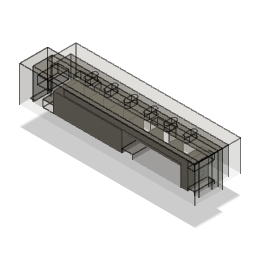
Ramp action bite sensor (Autodesk Fusion 360 design; units mm, degrees)
Autodesk Fusion 360 part; units mm, degrees
note: some values were not read from the file. Chosen so that the rebuilt part matches the saved one: which bodies a step acts on; which face or edge a step refers to. Set by a fixed rule: which sketch regions a step uses.
sketch "Sketch1" plane through (0, 0, 0) normal (0, 0, 1) x (1, 0, 0)
  line L0 (0, 0) -> (19.65, 0)
  line L1 (19.65, 0) -> (19.65, 6.7)
  line L2 (19.65, 6.7) -> (0, 6.7)
  line L3 (0, 6.7) -> (0, 0)
  dimension "d1" = 6.7
  dimension "d2" = 19.65
  constraint horizontal L0
  constraint vertical L1
  constraint horizontal L2
  constraint vertical L3
  constraint coincident L0.start L3.end
  measures "d1" distance of L0.start L2.end
  measures "d2" distance of L1 L3
extrude "Extrude1" add sketch "Sketch1" along normal blind 5.75 makes body 1
sketch "Sketch2" plane through (0, 0, 0) normal (-1, 0, 0) x (0, 0, 1)
  line L0 (0, 6.7) -> (0, 0)
  line L1 (0, 0) -> (5.75, 0)
  line L2 (5.75, 0) -> (5.75, 6.7)
  line L3 (5.75, 6.7) -> (0, 6.7)
  circle A0 centre (1.675, 0.4) radius 0.35
  circle A1 centre (2.875, 0.4) radius 0.35
  circle A2 centre (4.075, 0.4) radius 0.35
  line L4 (1.675, 0.4) -> (2.875, 0.4) construction
  line L5 (2.875, 0.4) -> (4.075, 0.4) construction
  line L6 (2.875, 0) -> (2.875, 1.1832) construction
  dimension "d5" = 0.7
  dimension "d6" = 1.2
  dimension "d7" = 0.4
  constraint equal A0 A1
  constraint equal A1 A2
  constraint coincident A0.centre L4.start
  constraint coincident A1.centre L4.end
  constraint parallel L1 L4
  constraint coincident A2.centre L5.end
  constraint parallel L4 L5
  constraint equal L4 L5
  constraint midpoint L1 L6.start
  constraint perpendicular L5 L6
  constraint coincident A1.centre L6
  measures "d5" diameter of A2
  measures "d6" distance of A0.centre A1.centre
  measures "d7" distance of L1 L5
extrude "Extrude2" add sketch "Sketch2" along normal blind 10 contours A0 | A1 | A2 bodies 1
sketch "Sketch3" plane through (0, 0, 0) normal (-1, 0, 0) x (0, 0, 1)
  circle A0 centre (1.675, 0.4) radius 0.35
  circle A1 centre (4.075, 0.4) radius 0.35
  line L0 (0, 6.7) -> (0, 0)
  line L1 (0, 0) -> (5.75, 0)
  line L2 (5.75, 0) -> (5.75, 6.7)
  line L3 (5.75, 6.7) -> (0, 6.7)
  line L4 (2.875, 6.7) -> (2.875, 2.6069) construction
  circle A2 centre (2.875, 4.5) radius 0.825
  circle A3 centre (2.875, 0.4) radius 0.35
  dimension "d10" = 1.65
  dimension "d11" = 4.5
  constraint midpoint L3 L4.start
  constraint perpendicular L3 L4
  constraint coincident L4 A2.centre
  measures "d10" diameter of A2
  measures "d11" distance of L1 A2.centre
extrude "Extrude3" cut sketch "Sketch3" against normal through all contours A2 bodies 1
sketch "Sketch4" plane through (0, 0, 0) normal (-1, 0, 0) x (0, 0, 1)
  circle A0 centre (2.875, 4.5) radius 0.825
  circle A1 centre (1.675, 0.4) radius 0.35
  circle A2 centre (4.075, 0.4) radius 0.35
  line L0 (0, 6.7) -> (0, 0)
  line L1 (0, 0) -> (5.75, 0)
  line L2 (5.75, 0) -> (5.75, 6.7)
  line L3 (5.75, 6.7) -> (0, 6.7)
  circle A3 centre (2.875, 4.5) radius 0.8
  circle A4 centre (2.875, 0.4) radius 0.35
  dimension "d13" = 1.6
  constraint concentric A0 A3
  measures "d13" diameter of A3
extrude "Extrude4" add sketch "Sketch4" along normal blind 0.4 and the other way blind 40 separate body contours A3 makes body 2
copy_body "Body->Comp1" bodies 1 removing the originals makes body 3 in component "Linear pot body"
copy_body "Body->Comp2" bodies 2 removing the originals makes body 4 in component "Linear pot shaft"
sketch "Sketch5" plane through (0, 0, 0) normal (0, 0, -1) x (-1, 0, 0)
  line L0 (0, 0) -> (0, 6.7)
  line L1 (0, 6.7) -> (-19.65, 6.7)
  line L2 (-19.65, 6.7) -> (-19.65, 0)
  line L3 (-19.65, 0) -> (0, 0)
  line L4 (1, -0.25) -> (1, -1.9)
  line L5 (1, -1.9) -> (-34.65, -1.9)
  line L6 (-34.65, -1.9) -> (-34.65, 8.6)
  line L7 (-34.65, 8.6) -> (1, 8.6)
  line L8 (1, 8.6) -> (1, 6.95)
  line L9 (1, 6.95) -> (-32.65, 6.95)
  line L10 (-32.65, 6.95) -> (-32.65, -0.25)
  line L11 (-32.65, -0.25) -> (1, -0.25)
  dimension "d26" = 0.25
  dimension "d27" = 0.25
  dimension "d28" = 1.65
  dimension "d29" = 1.65
  dimension "d30" = 13
  dimension "d31" = 2
  dimension "d34" = 1
  constraint perpendicular L3 L4
  constraint perpendicular L4 L5
  constraint perpendicular L5 L6
  constraint perpendicular L6 L7
  constraint perpendicular L5 L8
  constraint perpendicular L8 L9
  constraint perpendicular L5 L10
  constraint perpendicular L4 L11
  constraint collinear L4 L8
  measures "d26" distance of L3 L11
  measures "d27" distance of L1 L9
  measures "d28" distance of L5 L11
  measures "d29" distance of L7 L9
  measures "d30" distance of L2 L10
  measures "d31" distance of L6 L10
  measures "d34" distance of L0 L8
extrude "Extrude5" add sketch "Sketch5" against normal up to surface (5.75 mm away) separate body contours L4 L5 L6 L7 L8 L9 L10 L11 makes body 5
sketch "Sketch6" plane through (0, 8.6, 0) normal (0, 1, 0) x (-1, 0, 0)
  line L0 (-34.65, 0) -> (1, 0)
  line L1 (1, 0) -> (1, 5.75)
  line L2 (1, 5.75) -> (-34.65, 5.75)
  line L3 (-34.65, 5.75) -> (-34.65, 0)
  line L4 (1, 0) -> (-3.5, 4.5)
  line L5 (-3.5, 4.5) -> (-4.7, 4.5)
  line L6 (-4.7, 4.5) -> (-4.7, 0)
  line L7 (-4.7, 0) -> (-9.2, 4.5)
  line L8 (-9.2, 4.5) -> (-10.4, 4.5)
  line L9 (-10.4, 4.5) -> (-10.4, 0)
  line L10 (-10.4, 0) -> (-14.9, 4.5)
  line L11 (-14.9, 4.5) -> (-16.1, 4.5)
  line L12 (-16.1, 4.5) -> (-16.1, 0)
  line L13 (-16.1, 0) -> (-20.6, 4.5)
  line L14 (-20.6, 4.5) -> (-21.8, 4.5)
  line L15 (-21.8, 4.5) -> (-21.8, 0)
  line L16 (-21.8, 0) -> (-26.3, 4.5)
  line L17 (-26.3, 4.5) -> (-27.5, 4.5)
  line L18 (-27.5, 4.5) -> (-27.5, 0)
  line L19 (-27.5, 0) -> (-31.829, 4.329)
  line L20 (-31.829, 4.329) -> (-33.029, 4.329)
  line L21 (-33.029, 4.329) -> (-33.029, 0)
  dimension "d35" = 4.5
  dimension "d36" = 135
  dimension "d38" = 1.2
  dimension "d42" = 1.2
  dimension "d58" = 5.7
  constraint coincident L0.end L1.start
  constraint perpendicular L1 L5
  constraint coincident L0 L6.end
  constraint perpendicular L0 L6
  constraint perpendicular L6 L8
  constraint coincident L0 L9.end
  constraint perpendicular L0 L9
  constraint perpendicular L9 L11
  constraint coincident L0 L12.end
  constraint perpendicular L0 L12
  constraint parallel L10 L13
  constraint perpendicular L12 L14
  constraint coincident L0 L15.end
  constraint perpendicular L0 L15
  constraint parallel L13 L16
  constraint perpendicular L15 L17
  constraint coincident L0 L18.end
  constraint perpendicular L0 L18
  constraint collinear L5 L8
  constraint collinear L8 L11
  constraint collinear L11 L14
  constraint collinear L14 L17
  constraint equal L5 L8
  constraint equal L8 L11
  constraint equal L11 L14
  constraint equal L14 L17
  constraint parallel L7 L10
  constraint parallel L4 L7
  constraint perpendicular L18 L20
  constraint coincident L0 L21.end
  constraint perpendicular L0 L21
  constraint parallel L16 L19
  measures "d35" distance of L0 L5
  measures "d36" angle of L4 L5
  measures "d38" distance of L4.end L5.end
  measures "d42" distance of L19.end L20.end
  measures "d58" distance of L0.end L6.end
extrude "Extrude6" cut sketch "Sketch6" against normal through all contours L0 L19 L20 L21 | L0 L16 L17 L18 | L0 L13 L14 L15 | L0 L4 L5 L6 | L0 L10 L11 L12 | L0 L7 L8 L9 bodies 5
sketch "Sketch7" plane through (0, 0, 0) normal (0, 0, -1) x (-1, 0, 0)
  line L0 (0, 0) -> (0, 6.7)
  line L1 (0, 6.7) -> (-19.65, 6.7)
  line L2 (-19.65, 6.7) -> (-19.65, 0)
  line L3 (-19.65, 0) -> (0, 0)
  line L4 (4.7, 8.75) -> (-40.7, 8.75)
  line L5 (-40.7, 8.75) -> (-40.7, -2.05)
  line L6 (-40.7, -2.05) -> (4.7, -2.05)
  line L7 (4.7, -2.05) -> (4.7, 8.75)
  line L8 (-27.5, 8.6) -> (-26.3, 8.6)
  line L9 (-21.8, -1.9) -> (-26.3, -1.9)
  line L10 (4.2, 3.7) -> (4.2, 5.3)
  line L11 (-36.2, 5.3) -> (-36.2, 3.7)
  line L12 (-41.7, -3.05) -> (5.7, -3.05)
  line L13 (5.7, -3.05) -> (5.7, 9.75)
  line L14 (5.7, 9.75) -> (-41.7, 9.75)
  line L15 (-41.7, 9.75) -> (-41.7, -3.05)
  dimension "d44" = 0.15
  dimension "d45" = 0.15
  dimension "d46" = 0.5
  dimension "d47" = 4.5
  dimension "d48" = 1
  constraint horizontal L4
  constraint vertical L5
  constraint horizontal L6
  constraint vertical L7
  measures "d44" distance of L4 L8
  measures "d45" distance of L6 L9
  measures "d46" distance of L7 L10
  measures "d47" distance of L5 L11
extrude "Extrude7" add sketch "Sketch7" along normal blind 2.5 and the other way up to surface (5.75 mm away) separate body contours L12 L13 L14 L15 makes body 6
sketch "Sketch8" plane through (0, 8.75, 0) normal (0, -1, 0) x (1, 0, 0)
  line L0 (-4.7, 5.75) -> (-4.7, -2.5)
  line L1 (-4.7, -2.5) -> (40.7, -2.5)
  line L2 (40.7, -2.5) -> (40.7, 5.75)
  line L3 (40.7, 5.75) -> (-4.7, 5.75)
  circle A0 centre (32.2034, 3.5144) radius 0.75
  line L4 (32.2034, 3.5144) -> (32.2034, 1.5144) construction
  circle A1 centre (32.2034, 1.5144) radius 0.75
  line L5 (31.4534, 1.5144) -> (31.4534, 3.5144)
  line L6 (32.9534, 3.5144) -> (32.9534, 1.5144)
  dimension "d54" = 1.5
  dimension "d55" = 2
  constraint coincident A0.centre L4.start
  constraint perpendicular L1 L4
  constraint coincident L4.end A1.centre
  constraint equal A0 A1
  constraint coincident A0 L5.end
  constraint tangent A0 L5
  constraint tangent A1 L6
  constraint tangent A0 L6
  constraint coincident A0 L6.start
  constraint coincident A1 L5.start
  constraint tangent A1 L5
  constraint coincident A1 L6.end
  measures "d54" diameter of A0
  measures "d55" distance of A0.centre L4.end
extrude "Extrude8" add sketch "Sketch8" along normal blind 1.5 contours A0 | A0 A1 L5 L6 | A1 bodies 5 6
extrude "Extrude9" add sketch "Sketch8" against normal blind 1.75 from surface at 10.8 contours A0 | A0 A1 L5 L6 | A1 bodies 6
pattern_linear "R-Pattern1" count 6 spacing 5.7 along (-1, 0, 0) of "Extrude9"
pattern_linear "R-Pattern2" count 6 spacing 5.7 along (-1, 0, 0) of "Extrude8"
copy_body "Body->Comp3" bodies 6 removing the originals makes body 7 in component "Upper shell"
copy_body "Body->Comp5" bodies 5 removing the originals makes body 8 in component "Slider"
ref_plane "WorkPlane1" through (31.4534, 8, 3.5144) normal (-0.707107, 0, 0.707107) x (0, -1, 0) in component "Upper shell"
sketch "Sketch1 (2)" plane through (31.4534, 8, 3.5144) normal (-0.707107, 0, 0.707107) x (0, -1, 0) in component "Upper shell"
  line L0 (0, 0) -> (0, 0.75) construction
  dimension "d111" = 0.75
  constraint coincident L0.start origin
  constraint vertical L0
  measures "d111" distance of L0.start L0.end
sketch "Sketch2 (2)" plane through (0, 0, -2.5) normal (0, 0, -1) x (-1, 0, 0) in component "Upper shell"
  line L0 (4.7, 8.75) -> (4.7, -2.05)
  line L1 (4.7, -2.05) -> (-40.7, -2.05)
  line L2 (-40.7, -2.05) -> (-40.7, 8.75)
  line L3 (-40.7, 8.75) -> (4.7, 8.75)
  line L4 (-41.7, 9.75) -> (-41.7, -3.05)
  line L5 (-41.7, -3.05) -> (5.7, -3.05)
  line L6 (5.7, -3.05) -> (5.7, 9.75)
  line L7 (5.7, 9.75) -> (-41.7, 9.75)
extrude "Extrude1'" add sketch "Sketch2 (2)" against normal blind 2.5 contours L0 L1 L2 L3 bodies 7 in component "Upper shell"
sketch "Sketch9" plane through (0.75, 0, 5.75) normal (0, 0, 1) x (1, 0, 0)
  line L0 (-0.75, 6.95) -> (32.9, 6.95)
  line L1 (32.9, 6.95) -> (32.9, -0.25)
  line L2 (32.9, -0.25) -> (-0.75, -0.25)
  line L3 (-0.75, -0.25) -> (-0.75, -1.9)
  line L4 (-0.75, -1.9) -> (34.9, -1.9)
  line L5 (34.9, -1.9) -> (34.9, 8.6)
  line L6 (34.9, 8.6) -> (-0.75, 8.6)
  line L7 (-0.75, 8.6) -> (-0.75, 6.95)
  line L8 (39.95, -2.05) -> (-5.45, -2.05)
  line L9 (-5.45, -2.05) -> (-5.45, 8.75)
  line L10 (-5.45, 8.75) -> (39.95, 8.75)
  line L11 (39.95, 8.75) -> (39.95, -2.05)
  line L12 (-6.45, -3.05) -> (40.95, -3.05)
  line L13 (40.95, -3.05) -> (40.95, 9.75)
  line L14 (40.95, 9.75) -> (-6.45, 9.75)
  line L15 (-6.45, 9.75) -> (-6.45, -3.05)
extrude "Extrude10" add sketch "Sketch9" along normal blind 2.5 from surface at 0.02 separate body contours L0 L1 L2 L3 L4 L5 L6 L7 | L8 L9 L10 L11 | L12 L13 L14 L15 makes body 9
copy_body "Body->Comp6" bodies 9 removing the originals makes body 10 in component "Lower shell"
sketch "Sketch1 (3)" plane through (0, 0, 5.77) normal (0, 0, -1) x (-1, 0, 0) in component "Lower shell"
  line L0 (5.7, -3.05) -> (5.7, 9.75)
  line L1 (5.7, 9.75) -> (-41.7, 9.75)
  line L2 (-41.7, 9.75) -> (-41.7, -3.05)
  line L3 (-41.7, -3.05) -> (5.7, -3.05)
  line L4 (0.05, 3.1259) -> (3.05, 3.1259)
  line L5 (3.05, 3.1259) -> (3.05, 1.1259)
  line L6 (3.05, 1.1259) -> (0.05, 1.1259)
  line L7 (0.05, 1.1259) -> (0.05, 3.1259)
  line L8 (0, 6.7) -> (0, 0)
  line L9 (-19.7, 0.3387) -> (-22.8085, 0.3387)
  line L10 (-22.8085, 0.3387) -> (-22.8085, 2.2038)
  line L11 (-22.8085, 2.2038) -> (-19.7, 2.2038)
  line L12 (-19.7, 2.2038) -> (-19.7, 0.3387)
  line L13 (-19.65, 0) -> (-19.65, 6.7)
  dimension "d129" = 0.05
  dimension "d130" = 3
  dimension "d131" = 2
  dimension "d143" = 0.05
  constraint horizontal L4
  constraint vertical L5
  constraint horizontal L6
  constraint vertical L7
  constraint horizontal L9
  constraint vertical L10
  constraint horizontal L11
  constraint vertical L12
  measures "d129" distance of L7 L8
  measures "d130" distance of L5 L7
  measures "d131" distance of L4 L6
  measures "d143" distance of L12 L13
extrude "Extrude1''" add sketch "Sketch1 (3)" along normal up to surface (7.27 mm away) contours L4 L5 L6 L7 | L9 L10 L11 L12 bodies 10 in component "Lower shell"
sketch "Sketch2 (3)" plane through (-0.05, 0, 0) normal (1, 0, 0) x (0, 0, -1) in component "Lower shell"
  line L0 (1.5, 1.1259) -> (1.5, 3.1259)
  line L1 (1.5, 3.1259) -> (-5.77, 3.1259)
  line L2 (-5.77, 3.1259) -> (-5.77, 1.1259)
  line L3 (-5.77, 1.1259) -> (1.5, 1.1259)
  line L4 (1.5, 1.1259) -> (0, 1.1259)
  line L5 (0, 1.1259) -> (0, 3.1259)
  line L6 (0, 3.1259) -> (1.5, 3.1259)
  line L7 (1.5, 3.1259) -> (1.5, 1.1259)
  dimension "d134" = 1.5
  constraint horizontal L4
  constraint vertical L5
  constraint horizontal L6
  constraint vertical L7
  constraint coincident L1 L5.end
  constraint coincident L0.start L3.end
  measures "d134" distance of L5 L7
extrude "Extrude2'" add sketch "Sketch2 (3)" along normal blind 1.2 contours L0 L1 L3 L4 L5 L6 L7 bodies 10 in component "Lower shell"
sketch "Sketch3 (2)" plane through (0, 0, -2.5) normal (0, 0, -1) x (-1, 0, 0) in component "Upper shell"
  line L0 (-41.7, 9.75) -> (-41.7, -3.05)
  line L1 (-41.7, -3.05) -> (5.7, -3.05)
  line L2 (5.7, -3.05) -> (5.7, 9.75)
  line L3 (5.7, 9.75) -> (-41.7, 9.75)
  line L4 (-2.0163, 4.007) -> (3.8111, 4.007)
  line L5 (3.8111, 4.007) -> (3.8111, 0.2402)
  line L6 (3.8111, 0.2402) -> (-2.0163, 0.2402)
  line L7 (-2.0163, 0.2402) -> (-2.0163, 4.007)
  line L8 (-23.5837, 3.4089) -> (-18.248, 3.4089)
  line L9 (-18.248, 3.4089) -> (-18.248, -0.2119)
  line L10 (-18.248, -0.2119) -> (-23.5837, -0.2119)
  line L11 (-23.5837, -0.2119) -> (-23.5837, 3.4089)
  constraint horizontal L4
  constraint vertical L5
  constraint horizontal L6
  constraint vertical L7
  constraint horizontal L8
  constraint vertical L9
  constraint horizontal L10
  constraint vertical L11
extrude "Extrude2''" cut sketch "Sketch3 (2)" against normal through all from surface at -0.5 contours L4 L5 L6 L7 | L8 L9 L10 L11 bodies 7 in component "Upper shell"
sketch "Sketch3 (3)" plane through (0, 0, 5.77) normal (0, 0, -1) x (-1, 0, 0) in component "Lower shell"
  line L0 (3.05, 3.1259) -> (3.05, 1.1259)
  line L1 (3.05, 1.1259) -> (0.05, 1.1259)
  line L2 (0.05, 1.1259) -> (0.05, 3.1259)
  line L3 (0.05, 3.1259) -> (3.05, 3.1259)
  line L4 (5.7, -3.05) -> (5.7, 9.75)
  line L5 (5.7, 9.75) -> (-41.7, 9.75)
  line L6 (-41.7, 9.75) -> (-41.7, -3.05)
  line L7 (-41.7, -3.05) -> (5.7, -3.05)
  line L8 (4.55, 8.4492) -> (1.3881, 8.4492)
  line L9 (1.3881, 8.4492) -> (1.3881, 6.0241)
  line L10 (1.3881, 6.0241) -> (4.55, 6.0241)
  line L11 (4.55, 6.0241) -> (4.55, 8.4492)
  line L12 (4.55, -1.8262) -> (1.3881, -1.8262)
  line L13 (1.3881, -1.8262) -> (1.3881, -0.1246)
  line L14 (1.3881, -0.1246) -> (4.55, -0.1246)
  line L15 (4.55, -0.1246) -> (4.55, -1.8262)
  line L16 (-40.55, 8.4885) -> (-38.5504, 8.4885)
  line L17 (-38.5504, 8.4885) -> (-38.5504, 6.8746)
  line L18 (-38.5504, 6.8746) -> (-40.55, 6.8746)
  line L19 (-40.55, 6.8746) -> (-40.55, 8.4885)
  line L20 (-40.55, -1.7379) -> (-38.5504, -1.7379)
  line L21 (-38.5504, -1.7379) -> (-38.5504, 1.7763)
  line L22 (-38.5504, 1.7763) -> (-40.55, 1.7763)
  line L23 (-40.55, 1.7763) -> (-40.55, -1.7379)
  line L24 (-40.7, -2.05) -> (-40.7, 8.75)
  line L25 (4.7, 8.75) -> (4.7, -2.05)
  line L26 (-22.8085, 0.3387) -> (-22.8085, 2.2038)
  line L27 (-22.8085, 2.2038) -> (-19.7, 2.2038)
  line L28 (-19.7, 2.2038) -> (-19.7, 0.3387)
  line L29 (-19.7, 0.3387) -> (-22.8085, 0.3387)
  dimension "d139" = 0.15
  dimension "d140" = 0.15
  constraint horizontal L8
  constraint vertical L9
  constraint horizontal L10
  constraint vertical L11
  constraint horizontal L12
  constraint vertical L13
  constraint horizontal L14
  constraint vertical L15
  constraint horizontal L16
  constraint vertical L17
  constraint horizontal L18
  constraint vertical L19
  constraint horizontal L20
  constraint vertical L21
  constraint horizontal L22
  constraint vertical L23
  constraint collinear L17 L21
  constraint collinear L19 L23
  constraint collinear L11 L15
  constraint collinear L9 L13
  measures "d139" distance of L23 L24
  measures "d140" distance of L11 L25
extrude "Extrude3'" add sketch "Sketch3 (3)" along normal blind 5.8 contours L8 L9 L10 L11 | L12 L13 L14 L15 | L16 L17 L18 L19 | L20 L21 L22 L23 bodies 10 in component "Lower shell"
sketch "Sketch4 (2)" plane through (19.7, 0, 0) normal (-1, 0, 0) x (0, 0, 1) in component "Lower shell"
  line L0 (-1.5, 2.2038) -> (-1.5, 0.3387)
  line L1 (-1.5, 0.3387) -> (5.77, 0.3387)
  line L2 (5.77, 0.3387) -> (5.77, 2.2038)
  line L3 (5.77, 2.2038) -> (-1.5, 2.2038)
  line L4 (-1.5, 0.3387) -> (-0.05, 0.3387)
  line L5 (-0.05, 0.3387) -> (-0.05, 2.2038)
  line L6 (-0.05, 2.2038) -> (-1.5, 2.2038)
  line L7 (-1.5, 2.2038) -> (-1.5, 0.3387)
  line L8 (0, 0) -> (0, 6.7)
  dimension "d144" = 0.05
  constraint horizontal L4
  constraint vertical L5
  constraint horizontal L6
  constraint vertical L7
  constraint coincident L3 L5.end
  constraint coincident L0.end L1.start
  measures "d144" distance of L5 L8
extrude "Extrude4'" add sketch "Sketch4 (2)" along normal blind 1 contours L0 L1 L3 L4 L5 L6 L7 bodies 10 in component "Lower shell"
chamfer "Chamfer1" distance 1 angle 45 2 edges at (18.7, 1.2712, -1.5) (1.15, 2.1259, -1.5) on bodies 10 in component "Lower shell"
sketch "Sketch4 (3)" plane through (-5.7, 0, 0) normal (-1, 0, 0) x (0, 0, 1) in component "Upper shell"
  line L0 (5.75, 9.75) -> (-2.5, 9.75)
  line L1 (-2.5, 9.75) -> (-2.5, -3.05)
  line L2 (-2.5, -3.05) -> (5.75, -3.05)
  line L3 (5.75, -3.05) -> (5.75, 9.75)
  circle A0 centre (1.8509, 0.4011) radius 0.5
  line L4 (1.8509, 0.9011) -> (6.1961, 0.9011)
  line L5 (1.8509, -0.0989) -> (6.1961, -0.0989)
  line L6 (6.1961, -0.0989) -> (6.1961, 0.9011)
  dimension "d148" = 1
  constraint coincident A0 L4.start
  constraint perpendicular L3 L4
  constraint coincident A0 L5.start
  constraint perpendicular L3 L5
  constraint perpendicular L4 L6
  constraint tangent A0 L4
  constraint tangent A0 L5
  measures "d148" diameter of A0
extrude "Extrude3''" cut sketch "Sketch4 (3)" against normal blind 1.6 contours L3 A0 L4 L5 | A0 bodies 7 in component "Upper shell"
sketch "Sketch5 (2)" plane through (0, 0, 8.27) normal (0, 0, 1) x (1, 0, 0) in component "Lower shell"
  line L0 (-5.7, 9.75) -> (-5.7, -3.05)
  line L1 (-5.7, -3.05) -> (41.7, -3.05)
  line L2 (41.7, -3.05) -> (41.7, 9.75)
  line L3 (41.7, 9.75) -> (-5.7, 9.75)
  line L4 (-5.9, -3.25) -> (41.9, -3.25)
  line L5 (41.9, -3.25) -> (41.9, 9.95)
  line L6 (41.9, 9.95) -> (-5.9, 9.95)
  line L7 (-5.9, 9.95) -> (-5.9, -3.25)
  line L8 (-7.2, -4.55) -> (43.2, -4.55)
  line L9 (43.2, -4.55) -> (43.2, 11.25)
  line L10 (43.2, 11.25) -> (-7.2, 11.25)
  line L11 (-7.2, 11.25) -> (-7.2, -4.55)
  dimension "d151" = 0.2
  dimension "d152" = 1.5
extrude "Extrude5'" add sketch "Sketch5 (2)" against normal up to surface (2.5 mm away) contours L4 L5 L6 L7 bodies 10 in component "Lower shell"
extrude "Extrude6'" add sketch "Sketch5 (2)" against normal blind 8 contours L8 L9 L10 L11 bodies 10 in component "Lower shell"
sketch "Sketch6 (2)" plane through (-7.2, 0, 0) normal (-1, 0, 0) x (0, 0, 1) in component "Lower shell"
  line L0 (8.27, -4.55) -> (8.27, 11.25)
  line L1 (8.27, 11.25) -> (0.27, 11.25)
  line L2 (0.27, 11.25) -> (0.27, -4.55)
  line L3 (0.27, -4.55) -> (8.27, -4.55)
  circle A0 centre (5.1839, 0.3732) radius 0.6326
  line L4 (5.1839, 0.3732) -> (5.1839, 1.0059) construction
  line L5 (5.1839, 0.3732) -> (5.1839, -0.2594) construction
  line L6 (5.1839, 1.0059) -> (-0.3685, 1.0059)
  line L7 (-0.3685, 1.0059) -> (-0.3685, -0.2594)
  line L8 (-0.3685, -0.2594) -> (5.1839, -0.2594)
  constraint coincident A0.centre L4.start
  constraint coincident A0 L4.end
  constraint vertical L4
  constraint coincident A0 L5.end
  constraint parallel L4 L5
  constraint tangent A0 L6
  constraint perpendicular L6 L7
  constraint tangent A0 L8
extrude "Extrude7'" cut sketch "Sketch6 (2)" against normal blind 1.5 contours L2 L6 L7 L8 | L2 A0 L6 L8 | A0 bodies 10 in component "Lower shell"
sketch "Sketch1 (4)" plane through (33.029, 0, 0) normal (-1, 0, 0) x (0, 0, 1) in component "Slider"
  line L0 (0, -1.9) -> (4.329, -1.9)
  line L1 (4.329, -1.9) -> (4.329, 8.6)
  line L2 (4.329, 8.6) -> (0, 8.6)
  line L3 (0, 8.6) -> (0, -1.9)
  circle A0 centre (2.875, 4.5) radius 0.8
  circle A1 centre (2.875, 4.5) radius 0.85
  dimension "d159" = 1.7
  constraint concentric A0 A1
  measures "d159" diameter of A1
extrude "Extrude1'''" cut sketch "Sketch1 (4)" against normal through all contours A0 | A1 bodies 8 in component "Slider"
sketch "Sketch10" plane through (0, 0, 8.27) normal (0, 0, 1) x (1, 0, 0)
  line L0 (-7.2, 11.25) -> (-7.2, -4.55)
  line L1 (-7.2, -4.55) -> (43.2, -4.55)
  line L2 (43.2, -4.55) -> (43.2, 11.25)
  line L3 (43.2, 11.25) -> (-7.2, 11.25)
  line L4 (-7.7, -5.05) -> (43.7, -5.05)
  line L5 (43.7, -5.05) -> (43.7, 11.75)
  line L6 (43.7, 11.75) -> (-7.7, 11.75)
  line L7 (-7.7, 11.75) -> (-7.7, -5.05)
  line L8 (-9.05, -6.4) -> (45.05, -6.4)
  line L9 (45.05, -6.4) -> (45.05, 13.1)
  line L10 (45.05, 13.1) -> (-9.05, 13.1)
  line L11 (-9.05, 13.1) -> (-9.05, -6.4)
  dimension "d161" = 0.5
  dimension "d162" = 1.85
extrude "Extrude11" add sketch "Sketch10" against normal blind 7.5 separate body contours L8 L9 L10 L11 makes body 11
sketch "Sketch11" plane through (0, 0, 8.27) normal (0, 0, 1) x (1, 0, 0)
  line L0 (-7.7, -5.05) -> (-7.7, 11.75)
  line L1 (-7.7, 11.75) -> (43.7, 11.75)
  line L2 (43.7, 11.75) -> (43.7, -5.05)
  line L3 (43.7, -5.05) -> (-7.7, -5.05)
  line L4 (-9.05, 13.1) -> (-9.05, -6.4)
  line L5 (-9.05, -6.4) -> (45.05, -6.4)
  line L6 (45.05, -6.4) -> (45.05, 13.1)
  line L7 (45.05, 13.1) -> (-9.05, 13.1)
extrude "Extrude12" add sketch "Sketch11" along normal blind 2.25 contours L0 L1 L2 L3 | L4 L5 L6 L7 bodies 11
fillet "Fillet1" radius 1.5 8 edges at (-9.05, 13.1, 5.645) (18, 13.1, 10.52) (-9.05, 3.35, 10.52) (45.05, 3.35, 10.52) (45.05, 13.1, 5.645) (18, -6.4, 10.52) (45.05, -6.4, 5.645) (-9.05, -6.4, 5.645) on bodies 11
sketch "Sketch12" plane through (0, 0, 10.52) normal (0, 0, 1) x (1, 0, 0)
  line L0 (-7.55, -4.9) -> (43.55, -4.9)
  line L1 (43.55, -4.9) -> (43.55, 11.6)
  line L2 (43.55, 11.6) -> (-7.55, 11.6)
  line L3 (-7.55, 11.6) -> (-7.55, -4.9)
  line L4 (-6.55, -3.9) -> (42.55, -3.9)
  line L5 (42.55, -3.9) -> (42.55, 10.6)
  line L6 (42.55, 10.6) -> (-6.55, 10.6)
  line L7 (-6.55, 10.6) -> (-6.55, -3.9)
  dimension "d169" = -1
extrude "Extrude13" cut sketch "Sketch12" against normal blind 1.5 contours L4 L5 L6 L7 bodies 11
fillet "Fillet2" radius 0.5 7 edges at (18, 11.75, 8.27) (-7.7, 11.75, 4.52) (43.7, 11.75, 4.52) (43.7, 3.35, 8.27) (18, -5.05, 8.27) (43.7, -5.05, 4.52) (-7.7, -5.05, 4.52) on bodies 11
sketch "Sketch13" plane through (0, 0, 0.77) normal (0, 0, -1) x (-1, 0, 0)
  line L0 (7.7, 11.25) -> (7.7, -4.55)
  arc A0 (7.2, -5.05) -> (7.7, -4.55) centre (7.2, -4.55) ccw
  line L1 (7.2, -5.05) -> (-43.2, -5.05)
  arc A1 (-43.7, -4.55) -> (-43.2, -5.05) centre (-43.2, -4.55) ccw
  line L2 (-43.7, -4.55) -> (-43.7, 11.25)
  arc A2 (-43.2, 11.75) -> (-43.7, 11.25) centre (-43.2, 11.25) ccw
  line L3 (-43.2, 11.75) -> (7.2, 11.75)
  arc A3 (7.7, 11.25) -> (7.2, 11.75) centre (7.2, 11.25) ccw
  arc A4 (-45.05, -4.9) -> (-43.55, -6.4) centre (-43.55, -4.9) ccw
  line L4 (-43.55, -6.4) -> (7.55, -6.4)
  arc A5 (7.55, -6.4) -> (9.05, -4.9) centre (7.55, -4.9) ccw
  line L5 (9.05, -4.9) -> (9.05, 11.6)
  arc A6 (9.05, 11.6) -> (7.55, 13.1) centre (7.55, 11.6) ccw
  line L6 (7.55, 13.1) -> (-43.55, 13.1)
  arc A7 (-43.55, 13.1) -> (-45.05, 11.6) centre (-43.55, 11.6) ccw
  line L7 (-45.05, 11.6) -> (-45.05, -4.9)
  line L8 (-56.0207, 25.3049) -> (19.3626, 25.3049)
  line L9 (19.3626, 25.3049) -> (19.3626, -22.1267)
  line L10 (19.3626, -22.1267) -> (-56.0207, -22.1267)
  line L11 (-56.0207, -22.1267) -> (-56.0207, 25.3049)
  constraint horizontal L8
  constraint vertical L9
  constraint horizontal L10
  constraint vertical L11
extrude "Extrude14" add sketch "Sketch13" along normal blind 14 from surface at -14 separate body contours L0 A0 L1 A1 L2 A2 L3 A3 | A4 L4 A5 L5 A6 L6 A7 L7 | L8 L9 L10 L11 makes body 12
combine "Combine1" operation cut target body 12 tool bodies 11 keep tools makes body 13 at (30.893, 9.4944, 14.77)
sketch "Sketch14" plane through (0, 0, 0.77) normal (0, 0, -1) x (-1, 0, 0)
  line L0 (-56.0207, -22.1267) -> (19.3626, -22.1267)
  line L1 (19.3626, -22.1267) -> (19.3626, 25.3049)
  line L2 (19.3626, 25.3049) -> (-56.0207, 25.3049)
  line L3 (-56.0207, 25.3049) -> (-56.0207, -22.1267)
  arc A0 (9.05, 11.6) -> (7.55, 13.1) centre (7.55, 11.6) ccw
  line L4 (9.05, 11.6) -> (9.05, -4.9)
  arc A1 (7.55, -6.4) -> (9.05, -4.9) centre (7.55, -4.9) ccw
  line L5 (7.55, -6.4) -> (-43.55, -6.4)
  arc A2 (-45.05, -4.9) -> (-43.55, -6.4) centre (-43.55, -4.9) ccw
  line L6 (-45.05, -4.9) -> (-45.05, 11.6)
  arc A3 (-43.55, 13.1) -> (-45.05, 11.6) centre (-43.55, 11.6) ccw
  line L7 (-43.55, 13.1) -> (7.55, 13.1)
  circle A4 centre (-49.9767, 19.1899) radius 3
  circle A5 centre (-18, -15.0407) radius 3
  circle A6 centre (11.9336, 19.1899) radius 3
  dimension "d177" = 6
  constraint equal A4 A5
  constraint equal A5 A6
  measures "d177" diameter of A4
extrude "Extrude15" cut sketch "Sketch14" against normal blind 5 draft -5 contours A4 | A5 | A6 bodies 13
sketch "Sketch15" plane through (0, 0, 0.77) normal (0, 0, -1) x (-1, 0, 0)
  circle A0 centre (-49.9767, 19.1899) radius 3
  circle A1 centre (-18, -15.0407) radius 3
  circle A2 centre (11.9336, 19.1899) radius 3
  line L0 (-56.0207, -22.1267) -> (19.3626, -22.1267)
  line L1 (19.3626, -22.1267) -> (19.3626, 25.3049)
  line L2 (19.3626, 25.3049) -> (-56.0207, 25.3049)
  line L3 (-56.0207, 25.3049) -> (-56.0207, -22.1267)
  arc A3 (9.05, 11.6) -> (7.55, 13.1) centre (7.55, 11.6) ccw
  line L4 (9.05, 11.6) -> (9.05, -4.9)
  arc A4 (7.55, -6.4) -> (9.05, -4.9) centre (7.55, -4.9) ccw
  line L5 (7.55, -6.4) -> (-43.55, -6.4)
  arc A5 (-45.05, -4.9) -> (-43.55, -6.4) centre (-43.55, -4.9) ccw
  line L6 (-45.05, -4.9) -> (-45.05, 11.6)
  arc A6 (-43.55, 13.1) -> (-45.05, 11.6) centre (-43.55, 11.6) ccw
  line L7 (-43.55, 13.1) -> (7.55, 13.1)
  line L8 (-56.0207, 25.3049) -> (19.3626, 25.3049)
  line L9 (19.3626, 25.3049) -> (19.3626, -22.1267)
  line L10 (19.3626, -22.1267) -> (-56.0207, -22.1267)
  line L11 (-56.0207, -22.1267) -> (-56.0207, 25.3049)
  constraint horizontal L8
  constraint vertical L9
  constraint horizontal L10
  constraint vertical L11
  constraint coincident L0.end L1.start
  constraint coincident L2.end L3.start
extrude "Extrude16" add sketch "Sketch15" along normal blind 5 and the other way blind 14 separate body contours A0 | A1 | A2 | L0 L1 L2 L3 L8 L9 L10 L11 | A3 L4 A4 L5 A5 L6 A6 L7 makes body 14
combine "Combine2" operation cut target body 14 tool bodies 13 keep tools
sketch "Sketch16" plane through (0, 0, 0.77) normal (0, 0, 1) x (1, 0, 0)
  circle A0 centre (49.9767, 19.1899) radius 3
  circle A1 centre (18, -15.0407) radius 3
  circle A2 centre (-11.9336, 19.1899) radius 3
  line L0 (-19.3626, -22.1267) -> (56.0207, -22.1267)
  line L1 (56.0207, -22.1267) -> (56.0207, 25.3049)
  line L2 (56.0207, 25.3049) -> (-19.3626, 25.3049)
  line L3 (-19.3626, 25.3049) -> (-19.3626, -22.1267)
  arc A3 (-7.55, 13.1) -> (-9.05, 11.6) centre (-7.55, 11.6) ccw
  line L4 (-7.55, 13.1) -> (43.55, 13.1)
  arc A4 (45.05, 11.6) -> (43.55, 13.1) centre (43.55, 11.6) ccw
  line L5 (45.05, 11.6) -> (45.05, -4.9)
  arc A5 (43.55, -6.4) -> (45.05, -4.9) centre (43.55, -4.9) ccw
  line L6 (43.55, -6.4) -> (-7.55, -6.4)
  arc A6 (-9.05, -4.9) -> (-7.55, -6.4) centre (-7.55, -4.9) ccw
  line L7 (-9.05, -4.9) -> (-9.05, 11.6)
  line L8 (-10.5525, 14.8669) -> (46.1838, 14.8669)
  line L9 (46.1838, 14.8669) -> (46.1838, -8.3434)
  line L10 (46.1838, -8.3434) -> (-10.5525, -8.3434)
  line L11 (-10.5525, -8.3434) -> (-10.5525, 14.8669)
  constraint horizontal L8
  constraint vertical L9
  constraint horizontal L10
  constraint vertical L11
extrude "Extrude17" cut sketch "Sketch16" along normal blind 10 contours A3 L4 A4 L5 A5 L6 A6 L7 | L8 L9 L10 L11 bodies 14
combine "Combine3" operation add target body 12 tool bodies 14
sketch "Sketch17" plane through (0, 0, 0.77) normal (0, 0, -1) x (-1, 0, 0)
  circle A0 centre (-49.9767, 19.1899) radius 3
  circle A1 centre (-18, -15.0407) radius 3
  circle A2 centre (11.9336, 19.1899) radius 3
  line L0 (-56.0207, -22.1267) -> (19.3626, -22.1267)
  line L1 (19.3626, -22.1267) -> (19.3626, 25.3049)
  line L2 (19.3626, 25.3049) -> (-56.0207, 25.3049)
  line L3 (-56.0207, 25.3049) -> (-56.0207, -22.1267)
  arc A3 (9.05, 11.6) -> (7.55, 13.1) centre (7.55, 11.6) ccw
  line L4 (9.05, 11.6) -> (9.05, -4.9)
  arc A4 (7.55, -6.4) -> (9.05, -4.9) centre (7.55, -4.9) ccw
  line L5 (7.55, -6.4) -> (-43.55, -6.4)
  arc A5 (-45.05, -4.9) -> (-43.55, -6.4) centre (-43.55, -4.9) ccw
  line L6 (-45.05, -4.9) -> (-45.05, 11.6)
  arc A6 (-43.55, 13.1) -> (-45.05, 11.6) centre (-43.55, 11.6) ccw
  line L7 (-43.55, 13.1) -> (7.55, 13.1)
  circle A7 centre (-49.9767, 19.1899) radius 3.1
  circle A8 centre (-18, -15.0407) radius 3.1
  circle A9 centre (11.9336, 19.1899) radius 3.1
  dimension "d187" = 0.1
  dimension "d188" = 0.1
  dimension "d189" = 0.1
extrude "Extrude18" cut sketch "Sketch17" against normal blind 6 draft -5 contours A0 | A1 | A2 | A7 | A8 | A9 bodies 13
component "Linear pot body" placed x (1, 0, 0) y (0, 1, 0) z (0, 0, 1) at (0, 0, 0)
component "Linear pot shaft" placed x (1, 0, 0) y (0, 0.690209, 0.72361) z (0, -0.72361, 0.690209) at (-4.1, 3.4744, -2.3656)
component "Upper shell" placed x (1, 0, 0) y (0, 1, 0) z (0, 0, 1) at (0, 0, -0.1645)
component "Slider" placed x (1, 0, 0) y (0, 1, 0) z (0, 0, 1) at (0.25, 0, 0)
component "Lower shell" placed x (1, 0, 0) y (0, 1, 0) z (0, 0, 1) at (0, 0, 0)
hidden bodies 11 12 13
named bodies: "silicone cover lower half", "Silicone mold upper half", "Silicone mold lower half (1)"
